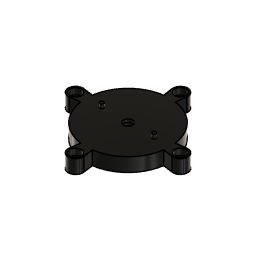
Pyramid_mirror_mount (Autodesk Fusion 360 design; units mm, degrees)
Autodesk Fusion 360 part; units mm, degrees
note: some values were not read from the file. Set by a fixed rule: which sketch regions a step uses.
sketch "Base" plane through (0, 0, 0) normal (0, 0, 1) x (1, 0, 0)
  circle A0 centre (0, 0) radius 40
  circle A1 centre (0, 0) radius 4.3
  line L0 (0, 0) -> (50, 0) construction
  circle A2 centre (25, 0) radius 1.75
  line L1 (0, 0) -> (0, 40) construction
  circle A3 centre (-25, 0) radius 1.75
  circle A4 centre (50, 0) radius 3.2
  circle A5 centre (0, 0) radius 10
  line L2 (7.0711, -7.0711) -> (28.2843, -28.2843)
  line L3 (7.0711, -7.0711) -> (0, 0) construction
  line L4 (7.0711, 7.0711) -> (3.0406, 3.0406)
  line L5 (7.0711, -7.0711) -> (3.0406, -3.0406)
  line L6 (7.0711, 7.0711) -> (28.2843, 28.2843)
  circle A6 centre (50, 0) radius 7
  line L7 (49.02, 6.9311) -> (39.6061, 5.6)
  line L8 (39.6061, 5.6) -> (0, 0) construction
  line L9 (49.02, -6.9311) -> (39.6061, -5.6)
  circle A7 centre (50, 0) radius 5.5
  dimension "d1" = 80
  dimension "d4" = 8.6
  dimension "d8" = 25
  dimension "d9" = 3.5
  dimension "d13" = 6.4
  dimension "d21" = 20
  dimension "d49" = 14
  dimension "d50" = 45
  dimension "d51" = 50
  dimension "d52" = 11
  constraint coincident A0.centre A1.centre
  constraint horizontal L0
  constraint coincident A0 L1.end
  constraint perpendicular L0 L1
  constraint coincident L0 A2.centre
  constraint symmetric A2 L1 A3
  constraint coincident A0 L7.end
  constraint coincident A5 L2.start
  constraint coincident A0 L2.end
  constraint collinear L2 L3
  constraint coincident A1 L4.end
  constraint symmetric L0 L4.start L2.start
  constraint symmetric L0 L4.end L5.end
  constraint symmetric L0 L2.start L4.start
  constraint symmetric L0 L2.end L6.end
  constraint collinear L2 L5
  constraint concentric A4 A6
  constraint coincident L0.end A4.centre
  constraint coincident A6 L7.start
  constraint tangent A6 L7
  constraint collinear L7 L8
  constraint symmetric L0 L7.end L9.end
  constraint symmetric L0 L7.start L9.start
  constraint concentric A6 A7
  measures "d1" diameter of A0
  measures "d4" diameter of A1
  measures "d8" distance of A0.centre A2.centre
  measures "d9" diameter of A2
  measures "d13" diameter of A4
  measures "d21" diameter of A5
  measures "d49" diameter of A6
  measures "d50" angle of L0 L6
  measures "d51" distance of A0.centre L0.end
  measures "d52" diameter of A7
extrude "Extrude1" add sketch "Base" against normal blind 13 contours A0 A5 L2 L6 | A0 A6 L7 L9 | A6 | A2 | A7 picked at (21.3272, -10.7092) makes body 1
extrude "Extrude6" add sketch "Base" against normal blind 3 contours A1 A5 L4 L5 picked at (8.0592, -0.6222) bodies 1
extrude "Extrude7" cut sketch "Base" against normal blind 6 contours A7 bodies 1
pattern_circular "C-Pattern2" count 4 over 360 about axis through (0, 0, 1.75) along (0, 0, 1) of bodies 1 makes body 2 at (0.1023, 27.8337, 0) makes body 3 at (-27.8337, 0.1023, 0) makes body 4 at (-0.1023, -27.8337, 0)
extrude "Extrude5" add sketch "Base" along normal blind 4 separate body contours A2 | A3 makes body 5 at (26.7478, -0.0872, 2.6667) makes body 6 at (-23.2522, -0.0872, 2.6667)
combine "Combine1" operation add target body 1 tool bodies 6 5 2 3 4
copy_body "Body->Comp1" bodies 1 removing the originals makes body 7 in component "Mirror_Pyramid_Mount"
component "Mirror_Pyramid_Mount" placed x (1, 0, 0) y (0, 1, 0) z (0, 0, 1) at (0, 0, 0)
equation "d51 = ( 2 * 25 ) * 1 mm"
